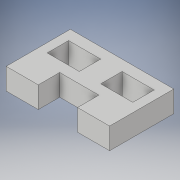
# Autodesk Inventor part: thumper-bumper-sidewall2-v3
Saved by Autodesk Inventor 2017 (Build 210142000, 142)
## iProperties
Created: 2017-02-22
Part Number: thumper-bumper-sidewall2-v3
Material: Generic
Document SubType Name: Modeling
Designer: John
Density: 1 g/cm^3
Appearance: Default
Author: John
Autodesk Inventor part; units mm, degrees
ref_plane "YZ Plane" through (0, 0, 0) normal (1, 0, 0) x (0, 1, 0)
ref_plane "XZ Plane" through (0, 0, 0) normal (0, 1, 0) x (-1, 0, 0)
ref_plane "XY Plane" through (0, 0, 0) normal (0, 0, 1) x (1, 0, 0)
sketch "Sketch1" plane through (0, 0, 0) normal (0, 1, 0) x (-1, 0, 0)
  line L0 (11.1299, 50.0199) -> (11.1299, 62.0199)
  line L1 (-17.8701, 62.0199) -> (-17.8701, 50.0199)
  line L2 (-17.8701, 50.0199) -> (-3.3701, 50.0199)
  line L3 (-3.3701, 50.0199) -> (-3.3701, 62.0199) construction
  line L4 (-17.8701, 56.0199) -> (-3.3701, 56.0199) construction
  line L5 (-17.8701, 62.0199) -> (11.1299, 62.0199)
  line L6 (-17.8701, 62.0199) -> (-8.8701, 62.0199)
  line L7 (-8.8701, 62.0199) -> (-8.8701, 68.0199)
  line L8 (-8.8701, 68.0199) -> (-17.8701, 68.0199)
  line L9 (-17.8701, 68.0199) -> (-17.8701, 62.0199)
  line L10 (11.1299, 62.0199) -> (2.1299, 62.0199)
  line L11 (2.1299, 62.0199) -> (2.1299, 68.0199)
  line L12 (2.1299, 68.0199) -> (11.1299, 68.0199)
  line L13 (11.1299, 68.0199) -> (11.1299, 62.0199)
  line L14 (-3.3701, 56.0199) -> (11.1299, 56.0199) construction
  line L15 (-3.3701, 50.0199) -> (11.1299, 50.0199)
  line L16 (-0.3701, 59.0199) -> (8.6299, 59.0199)
  line L17 (8.6299, 59.0199) -> (8.6299, 53.0199)
  line L18 (8.6299, 53.0199) -> (-0.3701, 53.0199)
  line L19 (-0.3701, 53.0199) -> (-0.3701, 59.0199)
  line L20 (-0.3701, 59.0199) -> (8.6299, 53.0199) construction
  line L21 (8.6299, 59.0199) -> (-0.3701, 53.0199) construction
  line L22 (-6.3701, 59.0199) -> (-15.3701, 59.0199)
  line L23 (-15.3701, 59.0199) -> (-15.3701, 53.0199)
  line L24 (-15.3701, 53.0199) -> (-6.3701, 53.0199)
  line L25 (-6.3701, 53.0199) -> (-6.3701, 59.0199)
  line L26 (-6.3701, 59.0199) -> (-15.3701, 53.0199) construction
  line L27 (-15.3701, 59.0199) -> (-6.3701, 53.0199) construction
  point P0 (4.1299, 56.0199)
  point P1 (-10.8701, 56.0199)
  dimension "d0" = 29
  dimension "d1" = 12
  dimension "d18" = 9
  dimension "d19" = 6
  dimension "d20" = 14.5
  dimension "d61" = 9
  dimension "d62" = 6
  dimension "d63" = 6
  dimension "d64" = 3
  constraints: 56 end point, 9 symmetric about line, 7 midpoint, 6 parallel, 5 horizontal, 2 equal length, 2 perpendicular, 2 point on line, 1 vertical
  measures "d0" distance of L1.start L0.end
  measures "d1" distance of L0.end L0.start
  measures "d18" distance of L8.end L7.end
  measures "d19" distance of L7.end L6.end
  measures "d20" distance between parallel lines of L3 L9
  measures "d61" distance of L17.end L18.end
  measures "d62" distance of L16.end L17.end
  measures "d63" distance between parallel lines of L25 L19
  measures "d64" distance between parallel lines of L5 L16
extrude "Extrusion1" add sketch "Sketch1" along normal blind 6
body "Solid1"
